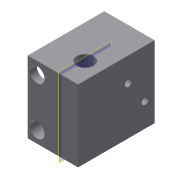
# Autodesk Inventor part: 30_CUBE_openXY_slider
Saved by Autodesk Inventor 2019 (Build 230136000, 136)
## iProperties
Created: 2020-01-07
Part Number: 30_CUBE_openXY_slider
Material: Generic
Document SubType Name: Modeling
Designer: diederichbenedict
Density: 1 g/cm^3
Appearance: Default
Author: diederichbenedict
Autodesk Inventor part; units mm, degrees
ref_plane "YZ Plane" through (0, 0, 0) normal (1, 0, 0) x (0, 1, 0)
ref_plane "XZ Plane" through (0, 0, 0) normal (0, 1, 0) x (-1, 0, 0)
sketch "Sketch1" plane through (0, 0, 0) normal (1, 0, 0) x (0, 1, 0)
  line L0 (0, 0) -> (30, 0)
  line L1 (30, 0) -> (30, 20)
  line L2 (30, 20) -> (0, 20)
  line L3 (0, 20) -> (0, 0)
  dimension "d0" = 30
  dimension "d1" = 20
  constraints: 8 end point, 2 parallel, 1 horizontal, 1 perpendicular
  measures "d0" distance of L2.end L1.end
  measures "d1" distance of L1.end L0.end
extrude "Extrusion1" add sketch "Sketch1" along normal blind 14
ref_plane "Work Plane1" through (7, 0, 0) normal (-1, 0, 0) x (0, 0, 1)
sketch "Sketch2" plane through (7, 0, 0) normal (-1, 0, 0) x (0, 0, 1)
  line L0 (20, 0) -> (0, 0) projected
  line L1 (10, 0) -> (10, 30)
  line L2 (0, 30) -> (20, 30) projected
  line L3 (3.8, 5.4) -> (16.2, 5.4)
  line L4 (16.2, 5.4) -> (16.2, 24.6)
  line L5 (16.2, 24.6) -> (3.8, 24.6)
  line L6 (3.8, 24.6) -> (3.8, 5.4)
  line L7 (3.8, 5.4) -> (16.2, 24.6) construction
  line L8 (16.2, 5.4) -> (3.8, 24.6) construction
  line L9 (10, 5.4) -> (6.5, 5.4)
  line L10 (6.5, 5.4) -> (6.5, 0)
  line L11 (6.5, 0) -> (10, 0)
  line L12 (10, 0) -> (10, 5.4)
  line L13 (10, 24.6) -> (6.5, 24.6)
  line L14 (6.5, 24.6) -> (6.5, 30)
  line L15 (6.5, 30) -> (10, 30)
  line L16 (10, 30) -> (10, 24.6)
  line L17 (10, 24.6) -> (3.8, 24.6)
  line L18 (3.8, 24.6) -> (3.8, 5.4)
  line L19 (3.8, 5.4) -> (10, 5.4)
  line L20 (10, 5.4) -> (10, 24.6)
  point P0 (10, 15)
  dimension "d5" = 12.4
  dimension "d6" = 19.2
  dimension "d7" = 3.5
  constraints: 38 end point, 8 parallel, 7 midpoint, 4 horizontal, 4 perpendicular, 3 point on line
  measures "d5" distance of L5.end L4.end
  measures "d6" distance of L4.end L3.end
  measures "d7" distance of L11.end L10.end
revolve "Revolution1" cut sketch "Sketch2" angle 360 about axis through (7, 0, 10) along (0, 1, 0) contours L0 L10 L3 L1 | L3 L6 L5 L1 | L5 L14 L2 L1
sketch "Sketch3" plane through (0, 0, 20) normal (0, 0, 1) x (1, 0, 0)
  line L0 (0, 30) -> (0, 0) projected
  line L1 (0, 0) -> (14, 0) projected
  line L2 (14, 30) -> (14, 0) projected
  line L3 (0, 30) -> (14, 30) projected
  line L4 (0, 0) -> (0, 30) projected
  line L5 (0, 0) -> (-7, 0)
  line L6 (-7, 0) -> (-7, 30)
  line L7 (-7, 30) -> (0, 30)
  line L8 (0, 30) -> (0, 0)
  line L9 (0, 30) -> (14, 30) projected
  circle A0 centre (-3.1, 5) radius 3.1
  line L10 (0, 30) -> (0, 0) projected
  circle A1 centre (-3.1, 25) radius 3.1
  dimension "d9" = 7
  dimension "d10" = 6.2
  dimension "d11" = 6.2
  dimension "d12" = 5
  dimension "d13" = 5
  constraints: 8 end point, 2 centre point, 2 parallel, 2 tangent, 1 horizontal, 1 perpendicular, 1 point on line
  measures "d9" distance of L6.end L7.end
  measures "d10" diameter of A0
  measures "d11" diameter of A1
  measures "d12" distance from line of A0.centre L5
  measures "d13" distance from line of A1.centre L7
extrude "Extrusion2" add sketch "Sketch3" against normal up to surface (20 mm away) contours L0 L5 L6 L7
sketch "Sketch4" plane through (-7, 0, 20) normal (-1, 0, 0) x (0, 0, 1)
  line L0 (-16.2, 24.6) -> (-16.2, 5.4) projected
  line L1 (-15, 24.5) -> (-5, 24.5) projected
  line L2 (-13.5, 24.6) -> (-6.5, 24.6) projected
  line L3 (-16.2, 5.4) -> (-3.8, 5.4) projected
  line L4 (-3.8, 24.6) -> (-3.8, 5.4) projected
  line L5 (-16.2, 24.6) -> (-3.8, 24.6) projected
  line L6 (-17, 25) -> (-3, 25)
  line L7 (-3, 25) -> (-3, 5)
  line L8 (-3, 5) -> (-17, 5)
  line L9 (-17, 5) -> (-17, 25)
  line L10 (-17, 25) -> (-3, 5) construction
  line L11 (-3, 25) -> (-17, 5) construction
  line L12 (-13.5, 30.2686) -> (-6.5, 30.2686)
  line L13 (-6.5, 30.2686) -> (-6.5, 25)
  line L14 (-6.5, 25) -> (-13.5, 25)
  line L15 (-13.5, 25) -> (-13.5, 30.2686)
  line L16 (-13.5, 30.2686) -> (-6.5, 25) construction
  line L17 (-6.5, 30.2686) -> (-13.5, 25) construction
  line L18 (-13.5, -0.71) -> (-6.5, -0.71)
  line L19 (-6.5, -0.71) -> (-6.5, 5)
  line L20 (-6.5, 5) -> (-13.5, 5)
  line L21 (-13.5, 5) -> (-13.5, -0.71)
  line L22 (-13.5, -0.71) -> (-6.5, 5) construction
  line L23 (-6.5, -0.71) -> (-13.5, 5) construction
  point P0 (-20, 0)
  point P1 (-10, 15)
  point P2 (-10, 27.6343)
  point P3 (-10, 2.145)
  dimension "d16" = 14
  dimension "d17" = 20
  dimension "d18" = 7
  constraints: 36 end point, 6 midpoint, 6 parallel, 3 horizontal, 3 perpendicular, 3 point on line
  measures "d16" distance of L7.end L8.end
  measures "d17" distance of L6.end L7.end
  measures "d18" distance of L13.end L14.end
extrude "Extrusion3" cut sketch "Sketch4" against normal blind 13 contours L5 L2 L4 L3 L0 | L6 L7 L8 L9
sketch "Sketch5" plane through (14, 0, 0) normal (0, 0, -1) x (-1, 0, 0)
  line L0 (21, 30) -> (0, 30) projected
  line L1 (0, 0) -> (0, 30) projected
  line L2 (21, 0) -> (0, 0) projected
  line L3 (21, 30) -> (21, 0) projected
  circle A0 centre (17.1, 25) radius 3.1 projected
  circle A1 centre (17.1, 5) radius 3.1 projected
  point P0 (14, 0)
ref_plane "Work Plane2" through (-3.5, -134.0004, -5) normal (0, 0, -1) x (0, 1, 0)
extrude "Extrusion4" add sketch "Sketch5" along normal blind 12
sketch "Sketch6" plane through (-7, 0, 20) normal (-1, 0, 0) x (0, 0, 1)
  point P0 (-20, 0)
sketch "Sketch7" plane through (-7, 0, 20) normal (-1, 0, 0) x (0, 0, 1)
  line L0 (-3, 5) -> (-17, 5) projected
  line L1 (-17, 5) -> (-17, 25) projected
  line L2 (-17, 25) -> (-3, 25) projected
  line L3 (-3, 25) -> (-3, 5) projected
  line L4 (0, 0) -> (-32, 0) projected
  line L5 (0, 30) -> (0, 0) projected
  line L6 (0, 30) -> (-32, 30) projected
  line L7 (-32, 0) -> (-32, 30) projected
  circle A0 centre (-28, 10) radius 1.4
  circle A1 centre (-21, 20) radius 1.4
  point P0 (-20, 0)
  dimension "d23" = 2.8
  dimension "d24" = 2.8
  dimension "d25" = 10
  dimension "d26" = 10
  dimension "d27" = 4
  dimension "d28" = 4
  constraints: 2 centre point
  measures "d23" diameter of A0
  measures "d24" diameter of A1
  measures "d25" distance from line of A1.centre L6
  measures "d26" distance from line of L4 A0.centre
  measures "d27" distance from line of L7 A0.centre
  measures "d28" distance from line of A1.centre L1
extrude "Extrusion5" cut sketch "Sketch7" against normal through all contours A0 | A1
sketch "Sketch8" plane through (14, 0, 20) normal (0, 0, 1) x (1, 0, 0)
  line L0 (-10, 99.8613) -> (-10, -100.1387)
  line L1 (-4, 99.8613) -> (-4, -100.1387)
  circle A0 centre (-7, 15) radius 1.4
  line L2 (-21, 0) -> (0, 0) projected
  point P0 (-14, 0)
  dimension "d31" = 2.8
  dimension "d32" = 15
  dimension "d33" = 3
  constraints: 4 end point, 2 vertical, 1 centre point, 4 other
  measures "d31" diameter of A0
  measures "d32" distance from line of L2 A0.centre
  measures "d33" distance from line of A0.centre L0
extrude "Extrusion6" cut sketch "Sketch8" against normal through all
body "Solid1"
